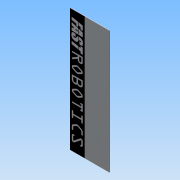
# Autodesk Inventor part: SideAccessPanel
Saved by Autodesk Inventor 2014 (Build 180170000, 170)
## iProperties
Created: 2014-01-06
Part Number: SideAccessPanel
Material: ABS Plastic
Document SubType Name: Modeling
Designer: davidgitz
Density: 1 g/cm^3
Appearance: Smooth - White
Author: davidgitz
Autodesk Inventor part; units mm, degrees
ref_plane "YZ Plane" through (0, 0, 0) normal (1, 0, 0) x (0, 1, 0)
ref_plane "XZ Plane" through (0, 0, 0) normal (0, 1, 0) x (-1, 0, 0)
ref_plane "XY Plane" through (0, 0, 0) normal (0, 0, 1) x (1, 0, 0)
sketch "Sketch1" plane through (0, 0, 0) normal (0, 0, 1) x (1, 0, 0)
  line L0 (-128.1216, 6.35) -> (-221.7407, 6.35) projected
  line L1 (-221.7407, -12.7) -> (-221.7407, 6.35) projected
  line L2 (-128.1216, -12.7) -> (-221.7407, -12.7) projected
  line L3 (-128.1216, -12.7) -> (-128.1216, 6.35) projected
  line L4 (-221.7407, -285.75) -> (-128.1216, -285.75) projected
  line L5 (-128.1216, -266.7) -> (-128.1216, -285.75) projected
  line L6 (-221.7407, -266.7) -> (-128.1216, -266.7) projected
  line L7 (-221.7407, -266.7) -> (-221.7407, -285.75) projected
  line L8 (-221.7407, 6.35) -> (-128.1216, 6.35)
  line L9 (-128.1216, 6.35) -> (-128.1216, -285.75)
  line L10 (-128.1216, -285.75) -> (-221.7407, -285.75)
  line L11 (-221.7407, -285.75) -> (-221.7407, 6.35)
  point P0 (0, 0)
  constraints: 8 end point, 2 parallel, 1 horizontal, 1 perpendicular
extrude "Extrusion1" add sketch "Sketch1" along normal blind 1.5875
sketch "Sketch2" plane through (0, 0, 1.5875) normal (0, 0, 1) x (1, 0, 0)
  line L0 (-128.1216, 6.35) -> (-221.7407, 6.35) projected
  line L1 (-186.5974, 6.35) -> (-186.5974, -285.75) construction
  line L2 (-186.5974, -285.75) -> (-221.7407, -285.75) construction
  line L3 (-221.7407, -285.75) -> (-221.7407, 6.35) construction
  line L4 (-221.7407, 6.35) -> (-186.5974, 6.35) construction
  point P0 (0, 0)
  constraints: 1 coincident, 1 point on line, 2 other
decal "Decal1"
body "Solid1"
